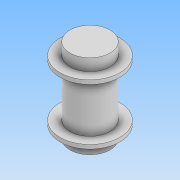
# Autodesk Inventor part: 特規趁套
Saved by Autodesk Inventor 2021 (Build 250183000, 183)
## iProperties
Created: 2025-12-12
Part Number: 特規趁套
Material: 一般
Document SubType Name: Modeling
Designer: User
Density: 1 g/cm^3
Appearance: 預設
Author: User
Autodesk Inventor part; units mm, degrees
ref_plane "YZ Plane" through (0, 0, 0) normal (1, 0, 0) x (0, 1, 0)
ref_plane "XZ Plane" through (0, 0, 0) normal (0, 1, 0) x (-1, 0, 0)
ref_plane "XY Plane" through (0, 0, 0) normal (0, 0, 1) x (1, 0, 0)
sketch "草圖1" plane through (0, 0, 0) normal (1, 0, 0) x (0, 1, 0)
  line L0 (0, 0) -> (10, 0)
  line L1 (10, 0) -> (10, -75)
  line L2 (10, -75) -> (0, -75)
  line L3 (0, -75) -> (0, 0)
  line L4 (140, 0) -> (150, 0)
  line L5 (150, 0) -> (150, -75)
  line L6 (150, -75) -> (140, -75)
  line L7 (140, -75) -> (140, 0)
  line L8 (10, 0) -> (140, 0)
  line L9 (140, 0) -> (140, -60)
  line L10 (10, -60) -> (10, 0)
  line L11 (-30, 0) -> (180, 0)
  line L12 (180, 0) -> (180, -50)
  line L13 (180, -50) -> (-30, -50)
  line L14 (-30, -50) -> (-30, 0)
  point P0 (0, -50)
  point P1 (10, -50)
  point P2 (140, -50)
  point P3 (150, -50)
  dimension "d0" = 10
  dimension "d1" = 150
  dimension "d2" = 150
  dimension "d3" = 10
  dimension "d5" = 100
  dimension "d6" = 210
  dimension "d7" = 30
  constraints: 30 end point, 7 parallel, 4 horizontal, 4 perpendicular, 2 horizontal alignment, 2 point on line, 1 coincident
  measures "d0" distance of L1.end L2.end
  measures "d1" diameter of L2 L0
  measures "d2" distance between parallel lines of L5 L3
  measures "d3" distance between parallel lines of L7 L5
  measures "d5" diameter of L13 L0
  measures "d6" distance of L12.end L13.end
  measures "d7" distance between parallel lines of L3 L14
revolve "迴轉1" add sketch "草圖1" angle 360 about axis through (0, 0, 0) along (0, 1, 0)
